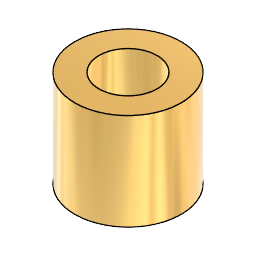
エレン_はさみ_mk1 v30 (Autodesk Fusion 360 archive; units mm, degrees)
design "インサートナット5.5*5mm"
Autodesk Fusion 360 part; units mm, degrees
note: some values were not read from the file. Set by a fixed rule: which face or edge a step refers to.
sketch "スケッチ1" plane through (0, 0, 0) normal (0, 0, 1) x (1, 0, 0)
  circle A0 centre (0, 0) radius 2.75
  circle A1 centre (0, 0) radius 1.5
  dimension "d1" = 5.5
  dimension "d2" = 3
  constraint coincident A0.centre A1.centre
  constraint concentric A0 A1
  measures "d1" diameter of A0
  measures "d2" diameter of A1
extrude "押し出し1" add sketch "スケッチ1" along normal blind 5

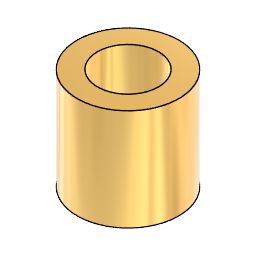
design "インサートナット5*5mm"
Autodesk Fusion 360 part; units mm, degrees
sketch "スケッチ1" plane through (0, 0, 0) normal (0, 0, 1) x (1, 0, 0)
  circle A0 centre (0, 0) radius 2.5
  circle A1 centre (0, 0) radius 1.5
  dimension "d1" = 5
  dimension "d2" = 3
  constraint coincident A0.centre A1.centre
  constraint concentric A0 A1
  measures "d1" diameter of A0
  measures "d2" diameter of A1
extrude "押し出し1" add sketch "スケッチ1" along normal blind 5

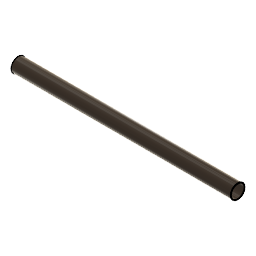
design "パイプ in30out33L500"
Autodesk Fusion 360 part; units mm, degrees
sketch "スケッチ2" plane through (0, 0, 0) normal (1, 0, 0) x (0, 1, 0)
  circle A0 centre (0, 0) radius 15
  circle A1 centre (0, 0) radius 16.5
  dimension "d1" = 30
  dimension "d2" = 33
  constraint coincident A0.centre A1.centre
  constraint concentric A0 A1
  measures "d1" diameter of A0
  measures "d2" diameter of A1
extrude "押し出し1" add sketch "スケッチ2" along normal blind 500

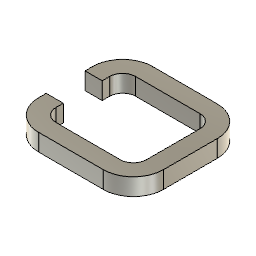
design "ring"
Autodesk Fusion 360 part; units mm, degrees
sketch "スケッチ1" plane through (0, 0, 0) normal (0, 0, 1) x (1, 0, 0)
  line L0 (10, 0) -> (40, 0)
  line L1 (50, 10) -> (50, 35)
  line L2 (40, 45) -> (10, 45)
  line L3 (0, 35) -> (0, 26)
  line L4 (0, 10) -> (0, 19)
  arc A0 (10, 45) -> (0, 35) centre (10, 35) ccw
  arc A1 (0, 10) -> (10, 0) centre (10, 10) ccw
  arc A2 (40, 0) -> (50, 10) centre (40, 10) ccw
  arc A3 (50, 35) -> (40, 45) centre (40, 35) ccw
  line L5 (0, 19) -> (0, 26) construction
  arc A4 (10, 49) -> (-4, 35) centre (10, 35) ccw
  line L6 (40, 49) -> (10, 49)
  arc A5 (54, 35) -> (40, 49) centre (40, 35) ccw
  line L7 (54, 10) -> (54, 35)
  arc A6 (40, -4) -> (54, 10) centre (40, 10) ccw
  line L8 (10, -4) -> (40, -4)
  arc A7 (-4, 10) -> (10, -4) centre (10, 10) ccw
  arc A8 (10, 41) -> (4, 35) centre (10, 35) ccw
  line L9 (40, 41) -> (10, 41)
  arc A9 (46, 35) -> (40, 41) centre (40, 35) ccw
  line L10 (46, 10) -> (46, 35)
  arc A10 (40, 4) -> (46, 10) centre (40, 10) ccw
  line L11 (10, 4) -> (40, 4)
  arc A11 (4, 10) -> (10, 4) centre (10, 10) ccw
  line L12 (4, 35) -> (4, 32.5)
  line L13 (4, 32.5) -> (-4, 32.5)
  line L14 (-4, 32.5) -> (-4, 35)
  line L15 (4, 10) -> (4, 12.5)
  line L16 (4, 12.5) -> (-4, 12.5)
  line L17 (-4, 12.5) -> (-4, 10)
  point P0 (50, 0)
  point P1 (0, 45)
  dimension "d1" = 50
  dimension "d2" = 45
  dimension "d3" = 19
  dimension "d4" = 19
  dimension "d5" = 10
  dimension "d8" = 4
  dimension "d9" = -4
  dimension "d16" = 2.5
  dimension "d17" = 2.5
  constraint horizontal L0
  constraint vertical L1
  constraint horizontal L2
  constraint perpendicular L2 L3
  constraint perpendicular L0 L4
  constraint coincident P1 L3
  constraint coincident P1 L2
  constraint tangent L3 A0
  constraint tangent L2 A0
  constraint coincident origin L4
  constraint coincident origin L0
  constraint tangent L4 A1
  constraint tangent L0 A1
  constraint equal A0 A1
  constraint coincident P0 L0
  constraint coincident P0 L1
  constraint tangent L0 A2
  constraint tangent L1 A2
  constraint equal A0 A2
  constraint tangent L1 A3
  constraint tangent L2 A3
  constraint equal A0 A3
  constraint parallel L3 L5
  constraint parallel L3 L12
  constraint perpendicular L12 L13
  constraint tangent A4 L14
  constraint vertical L15
  constraint perpendicular L4 L16
  constraint tangent A7 L17
  measures "d1" distance of origin P0
  measures "d2" distance of origin P1
  measures "d3" distance of P1 L3.end
  measures "d4" distance of origin L4.end
  measures "d5" radius of A0
  measures "d16" distance of A8.end L12.end
  measures "d17" distance of A11.start L15.end
extrude "押し出し1" add sketch "スケッチ1" along normal blind 8
extrude "押し出し4" add 2 faces at (-1.3333, 32.5, 2.6667) (2.6667, 32.5, 2.6667) along direction (0, -1, 0) blind 1
extrude "押し出し5" add 1 faces at (1.3333, 12.5, 2.6667) along direction (0, 1, 0) blind 1
equation "d3 = d4"
equation "d9 = -d8"

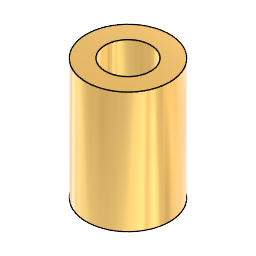
design "インサートナット5.5*8mm"
Autodesk Fusion 360 part; units mm, degrees
sketch "スケッチ1" plane through (0, 0, 0) normal (0, 0, 1) x (1, 0, 0)
  circle A0 centre (0, 0) radius 2.75
  circle A1 centre (0, 0) radius 1.5
  dimension "d1" = 5.5
  dimension "d2" = 3
  constraint coincident A0.centre A1.centre
  constraint concentric A0 A1
  measures "d1" diameter of A0
  measures "d2" diameter of A1
extrude "押し出し1" add sketch "スケッチ1" along normal blind 8
